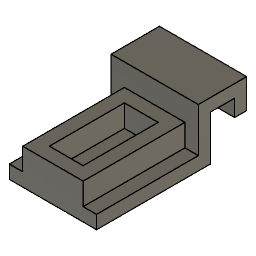
mount_ (Autodesk Fusion 360 design; units mm, degrees)
Autodesk Fusion 360 part; units mm, degrees
sketch "Sketch1" plane through (0, 0, 0) normal (0, 0, 1) x (1, 0, 0)
  line L0 (-41.91, -4.445) -> (41.91, -4.445)
  line L1 (41.91, -4.445) -> (41.91, 4.445)
  line L2 (41.91, 4.445) -> (-41.91, 4.445)
  line L3 (-41.91, 4.445) -> (-41.91, -4.445)
  line L4 (-41.91, 4.445) -> (41.91, -4.445) construction
  line L5 (41.91, 4.445) -> (-41.91, -4.445) construction
  dimension "d1" = 83.82
  dimension "d2" = 8.89
  constraint horizontal L0
  constraint vertical L1
  constraint horizontal L2
  constraint vertical L3
  constraint midpoint L5 origin
  measures "d1" distance of L0.start L0.end
  measures "d2" distance of L0.start L2.end
extrude "Extrude1" add sketch "Sketch1" along normal blind 4.7171 makes body 1
sketch "Sketch2" plane through (0, 0, 4.7171) normal (0, 0, 1) x (-1, 0, 0)
  line L0 (41.91, -4.445) -> (41.91, 4.445)
  line L1 (41.91, 4.445) -> (-41.91, 4.445)
  line L2 (-41.91, 4.445) -> (-41.91, -4.445)
  line L3 (-41.91, -4.445) -> (41.91, -4.445)
  line L4 (-41.91, -4.445) -> (41.91, -4.445)
  line L5 (41.91, -4.445) -> (41.91, -9.105)
  line L6 (41.91, -9.105) -> (-41.91, -9.105)
  line L7 (-41.91, -9.105) -> (-41.91, -4.445)
  line L8 (-41.91, -4.555) -> (41.91, -4.555)
  dimension "d5" = 4.66
  dimension "d34" = 0.11
  constraint horizontal L4
  constraint vertical L5
  constraint horizontal L6
  constraint vertical L7
  constraint coincident L2.end L3.start
  constraint vertical L0.start L5.end
  constraint coincident L7 L8.start
  constraint coincident L5 L8.end
  constraint perpendicular L5 L8
  measures "d5" distance of L2.end L6.end
  measures "d34" distance of L4 L8
extrude "Extrude2" add sketch "Sketch2" against normal blind 11.0067 separate body contours L5 L6 L7 L8 makes body 2
sketch "Sketch3" plane through (0, 0, 4.7171) normal (0, 0, 1) x (-1, 0, 0)
  line L0 (41.91, -4.445) -> (41.91, 4.445)
  line L1 (41.91, 4.445) -> (-41.91, 4.445)
  line L2 (-41.91, 4.445) -> (-41.91, -4.445)
  line L3 (-41.91, -9.105) -> (41.91, -9.105)
  line L4 (41.91, 4.445) -> (-41.91, 4.445)
  line L5 (-41.91, 4.445) -> (-41.91, 8.995)
  line L6 (-41.91, 8.995) -> (41.91, 8.995)
  line L7 (41.91, 8.995) -> (41.91, 4.445)
  line L8 (-41.91, -4.445) -> (41.91, -4.445)
  line L9 (-41.91, -4.555) -> (-41.91, -9.105)
  line L10 (41.91, -9.105) -> (41.91, -4.555)
  line L11 (41.91, -4.555) -> (-41.91, -4.555)
  dimension "d8" = 4.55
  constraint horizontal L4
  constraint vertical L5
  constraint horizontal L6
  constraint vertical L7
  constraint coincident L0.end L1.start
  constraint vertical L1.end L5.end
  measures "d8" distance of L0.end L6.end
extrude "Extrude3" add sketch "Sketch3" against normal blind 16.51 contours L1 L4 L5 L6 L7 bodies 1
ref_plane "WorkPlane1" through (0, -2.275, -11.7929) normal (0, 0, 1) x (1, 0, 0)
sketch "Sketch4" plane through (0, 0, -11.7929) normal (0, 0, 1) x (1, 0, 0)
  line L0 (41.91, -8.995) -> (-41.91, -8.995)
  line L1 (-41.91, -8.995) -> (41.91, -8.995)
  line L2 (41.91, -8.995) -> (41.91, -38.995)
  line L3 (41.91, -38.995) -> (-41.91, -38.995)
  line L4 (-41.91, -38.995) -> (-41.91, -8.995)
  dimension "d12" = 30
  constraint horizontal L1
  constraint vertical L2
  constraint horizontal L3
  constraint vertical L4
  constraint coincident L0.end L1.start
  constraint vertical L0.start L2.end
  measures "d12" distance of L0.end L3.end
extrude "Extrude4" add sketch "Sketch4" against normal blind 5 separate body makes body 3
sketch "Sketch5" plane through (0, 0, -11.7929) normal (0, 0, -1) x (1, 0, 0)
  line L0 (41.91, 8.995) -> (-41.91, 8.995)
  line L1 (-41.91, 8.995) -> (-41.91, 4.445)
  line L2 (-41.91, 4.445) -> (41.91, 4.445)
  line L3 (41.91, 4.445) -> (41.91, 8.995)
extrude "Extrude5" add sketch "Sketch5" along normal blind 5 bodies 1 3
extrude "Extrude6" add 1 faces at (13.97, -38.995, -13.4595) along direction (0, -1, 0) blind 8 on bodies 1 bodies 1
sketch "Sketch6" plane through (0, 0, -11.7929) normal (0, 0, 1) x (-1, 0, 0)
  line L0 (-41.91, 46.995) -> (-41.91, 8.995)
  line L1 (-41.91, 8.995) -> (41.91, 8.995)
  line L2 (41.91, 8.995) -> (41.91, 46.995)
  line L3 (6.3, 13.995) -> (-6.3, 13.995)
  line L4 (-6.3, 13.995) -> (-6.3, 41.995)
  line L5 (-6.3, 41.995) -> (6.3, 41.995)
  line L6 (6.3, 41.995) -> (6.3, 13.995)
  line L7 (6.3, 13.995) -> (-6.3, 41.995) construction
  line L8 (-6.3, 13.995) -> (6.3, 41.995) construction
  line L9 (-41.91, 8.995) -> (41.91, 8.995)
  line L10 (41.91, 46.995) -> (-41.91, 46.995)
  line L11 (11.3, 8.995) -> (-11.3, 8.995)
  line L12 (-11.3, 8.995) -> (-11.3, 46.995)
  line L13 (-11.3, 46.995) -> (11.3, 46.995)
  line L14 (11.3, 46.995) -> (11.3, 8.995)
  line L15 (0, 8.995) -> (0, 46.995) construction
  line L16 (16.3, 8.995) -> (-16.3, 8.995)
  line L17 (-16.3, 8.995) -> (-16.3, 46.995)
  line L18 (-16.3, 46.995) -> (16.3, 46.995)
  line L19 (16.3, 46.995) -> (16.3, 8.995)
  dimension "d17" = 12.6
  dimension "d18" = 28
  dimension "d22" = 5
  dimension "d23" = 5
  dimension "d24" = 5
  dimension "d25" = 5
  dimension "d26" = 5
  dimension "d27" = 25.61
  constraint horizontal L3
  constraint vertical L4
  constraint horizontal L5
  constraint vertical L6
  constraint horizontal L11
  constraint vertical L12
  constraint horizontal L13
  constraint vertical L14
  constraint coincident L10 L12.end
  constraint coincident L9 L11.start
  constraint midpoint L9 L15.start
  constraint midpoint L13 L15.end
  constraint perpendicular L13 L15
  constraint horizontal L16
  constraint vertical L17
  constraint horizontal L18
  constraint vertical L19
  constraint coincident L10 L17.end
  constraint coincident L1 L16.start
  measures "d17" distance of L3.start L3.end
  measures "d18" distance of L3.start L5.end
  measures "d22" distance of L5 L10
  measures "d23" distance of L4 L12
  measures "d24" distance of L6 L14
  measures "d25" distance of L14 L19
  measures "d26" distance of L12 L17
  measures "d27" distance of L2 L19
extrude "Extrude7" cut 1 faces at (-41.91, -20.145, -15.1262) along direction (1, 0, 0) blind 25.61 on bodies 1 bodies 1
extrude "Extrude8" cut 1 faces at (41.91, -20.145, -15.1262) along direction (-1, 0, 0) blind 25.61 on bodies 1 bodies 1
extrude "Extrude9" add sketch "Sketch6" along normal blind 8.25 contours L1 L9 L10 L11 L12 L13 L14 L16 L18 bodies 1
extrude "Extrude10" add 1 faces at (5.4333, 4.445, 1.5724) along direction (0, 1, 0) blind 0.11 on bodies 1 bodies 1 2
extrude "Extrude11" cut 1 faces at (41.91, 7.5883, 1.0483) along direction (-1, 0, 0) blind 25.61 on bodies 1 bodies 1
extrude "Extrude12" cut 1 faces at (-41.91, 6.0717, 1.0483) along direction (1, 0, 0) blind 25.61 on bodies 1 bodies 1
equation "d3 = ( 33.02 / 7 ) * 1 mm"
equation "d6 = ( ( -2 * 33.02 ) / 6 ) * 1 mm"
equation "d9 = ( -33.02 / 2 ) * 1 mm"
equation "d11 = ( -33.02 / 2 ) * 1 mm"
equation "d32 = ( 33 / 4 ) * 1 mm"
